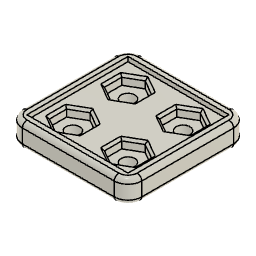
Foot_PartB_x6 (Autodesk Fusion 360 design; units mm, degrees)
Autodesk Fusion 360 part; units mm, degrees
sketch "Sketch1" plane through (0, 0, 0) normal (0, 0, 1) x (1, 0, 0)
  line L0 (0, 0) -> (26, 0)
  line L1 (26, 0) -> (26, 26)
  line L2 (26, 26) -> (0, 26)
  line L3 (0, 26) -> (0, 0)
  dimension "d1" = 26
  dimension "d2" = 26
  constraint horizontal L0
  constraint vertical L1
  constraint horizontal L2
  constraint vertical L3
  constraint coincident L0.start L3.end
  measures "d1" distance of L0.start L0.end
  measures "d2" distance of L0.start L2.end
extrude "Extrude1" add sketch "Sketch1" along normal blind 2
sketch "Sketch2" plane through (0, 0, 2) normal (0, 0, 1) x (-1, 0, 0)
  line L0 (0, -26) -> (0, 0)
  line L1 (0, 0) -> (-26, 0)
  line L2 (-26, 0) -> (-26, -26)
  line L3 (-26, -26) -> (0, -26)
  line L4 (-2, -24) -> (-24, -24)
  line L5 (-24, -24) -> (-24, -2)
  line L6 (-24, -2) -> (-2, -2)
  line L7 (-2, -2) -> (-2, -24)
  constraint horizontal L4
  constraint vertical L5
  constraint horizontal L6
  constraint vertical L7
extrude "Extrude2" add sketch "Sketch2" along normal blind 1.5
extrude "Extrude3" add 1 faces at (0.6667, 9.3333, 3.5) along direction (0, 0, 1) blind 2
extrude "Extrude4" add 1 faces at (9.3333, 16.6667, 2) along direction (0, 0, 1) blind 2
extrude "Extrude5" cut 1 faces at (0.6667, 9.3333, 5.5) along direction (0, 0, -1) blind 0.5
fillet "Fillet1" radius 3 4 edges at (0, 26, 2.5) (26, 26, 2.5) (0, 0, 2.5) (26, 0, 2.5)
fillet "Fillet2" radius 1 16 edges at (0, 13, 5) (0.8787, 25.1213, 5) (13, 26, 5) (25.1213, 25.1213, 5) (26, 13, 5) (25.1213, 0.8787, 5) (13, 0, 5) (0.8787, 0.8787, 5) (26, 13, 0) (25.1213, 25.1213, 0) (13, 26, 0) (0.8787, 25.1213, 0) (0, 13, 0) (0.8787, 0.8787, 0) (13, 0, 0) (25.1213, 0.8787, 0)
sketch "Sketch3" plane through (0, 0, 4) normal (0, 0, 1) x (-1, 0, 0)
  line L0 (-24, -2) -> (-24, -24)
  line L1 (-24, -24) -> (-2, -24)
  line L2 (-2, -24) -> (-2, -2)
  line L3 (-2, -2) -> (-24, -2)
  circle A0 centre (-7, -19) radius 1.5
  circle A1 centre (-19, -19) radius 1.5
  circle A2 centre (-19, -7) radius 1.5
  circle A3 centre (-7, -7) radius 1.5
  dimension "d16" = 3
  dimension "d17" = 3
  dimension "d18" = 3
  dimension "d19" = 3
  measures "d16" diameter of A0
  measures "d17" diameter of A1
  measures "d18" diameter of A2
  measures "d19" diameter of A3
extrude "Extrude6" cut sketch "Sketch3" against normal blind 4 contours A0 | A1 | A2 | A3
sketch "Sketch4" plane through (0, 0, 4) normal (0, 0, 1) x (-1, 0, 0)
  circle A0 centre (-7, -19) radius 1.5
  circle A1 centre (-7, -7) radius 1.5
  circle A2 centre (-19, -19) radius 1.5
  circle A3 centre (-19, -7) radius 1.5
  line L0 (-24, -2) -> (-24, -24)
  line L1 (-24, -24) -> (-2, -24)
  line L2 (-2, -24) -> (-2, -2)
  line L3 (-2, -2) -> (-24, -2)
  line L4 (-10.25, -20.8764) -> (-7, -22.7528)
  line L5 (-7, -22.7528) -> (-3.75, -20.8764)
  line L6 (-3.75, -20.8764) -> (-3.75, -17.1236)
  line L7 (-3.75, -17.1236) -> (-7, -15.2472)
  line L8 (-7, -15.2472) -> (-10.25, -17.1236)
  line L9 (-10.25, -17.1236) -> (-10.25, -20.8764)
  line L10 (-22.25, -20.8764) -> (-19, -22.7528)
  line L11 (-19, -22.7528) -> (-15.75, -20.8764)
  line L12 (-15.75, -20.8764) -> (-15.75, -17.1236)
  line L13 (-15.75, -17.1236) -> (-19, -15.2472)
  line L14 (-19, -15.2472) -> (-22.25, -17.1236)
  line L15 (-22.25, -17.1236) -> (-22.25, -20.8764)
  line L16 (-10.25, -8.8764) -> (-7, -10.7528)
  line L17 (-7, -10.7528) -> (-3.75, -8.8764)
  line L18 (-3.75, -8.8764) -> (-3.75, -5.1236)
  line L19 (-3.75, -5.1236) -> (-7, -3.2472)
  line L20 (-7, -3.2472) -> (-10.25, -5.1236)
  line L21 (-10.25, -5.1236) -> (-10.25, -8.8764)
  line L22 (-22.25, -8.8764) -> (-19, -10.7528)
  line L23 (-19, -10.7528) -> (-15.75, -8.8764)
  line L24 (-15.75, -8.8764) -> (-15.75, -5.1236)
  line L25 (-15.75, -5.1236) -> (-19, -3.2472)
  line L26 (-19, -3.2472) -> (-22.25, -5.1236)
  line L27 (-22.25, -5.1236) -> (-22.25, -8.8764)
  point P0 (-7, -19)
  point P1 (-19, -19)
  point P2 (-7, -7)
  point P3 (-19, -7)
  dimension "d22" = 3.25
  dimension "d23" = 3.25
  dimension "d24" = 3.25
  dimension "d25" = 3.25
  constraint coincident P0 A0.centre
  constraint coincident P1 A2.centre
  constraint coincident A1.centre P2
  constraint coincident P3 A3.centre
  measures "d22" distance of P0 L9
  measures "d23" distance of P1 L15
  measures "d24" distance of P2 L21
  measures "d25" distance of P3 L27
extrude "Extrude7" cut sketch "Sketch4" against normal blind 2 contours L4 L5 L6 L7 L8 L9 | L10 L11 L12 L13 L14 L15 | L16 L17 L18 L19 L20 L21 | L22 L23 L24 L25 L26 L27
chamfer "Chamfer1" distance 0.5 angle 45 24 edges at (8.625, 4.1854, 4) (5.375, 4.1854, 4) (3.75, 7, 4) (5.375, 9.8146, 4) (8.625, 9.8146, 4) (10.25, 7, 4) (8.625, 16.1854, 4) (5.375, 16.1854, 4) (3.75, 19, 4) (5.375, 21.8146, 4) (8.625, 21.8146, 4) (10.25, 19, 4) (17.375, 21.8146, 4) (15.75, 19, 4) (17.375, 16.1854, 4) (20.625, 16.1854, 4) (22.25, 19, 4) (20.625, 21.8146, 4) (17.375, 9.8146, 4) (15.75, 7, 4) (17.375, 4.1854, 4) (20.625, 4.1854, 4) (22.25, 7, 4) (20.625, 9.8146, 4)
